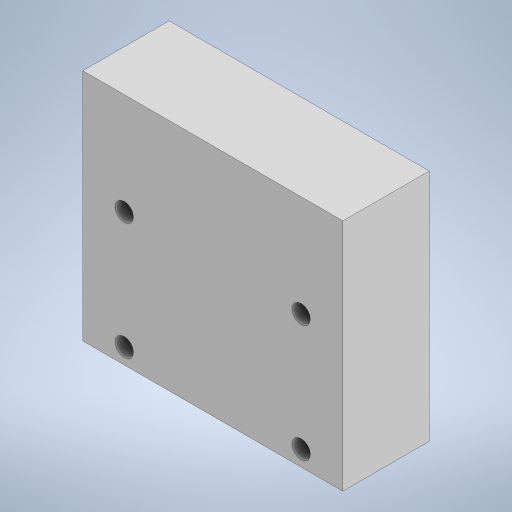
# Autodesk Inventor part: SUSTAINA-AUDIO-BOARD
Saved by Autodesk Inventor 2024.2 (Build 282272000, 272)
## iProperties
Created: 2024-06-01
Part Number: SUSTAINA-AUDIO-BOARD
Material: Generic
Document SubType Name: Modeling
Designer: Masato Kubotera
Density: 1 g/cm^3
Appearance: Default
Author: Masato Kubotera
Autodesk Inventor part; units mm, degrees
ref_plane "YZ Plane" through (0, 0, 0) normal (1, 0, 0) x (0, 1, 0)
ref_plane "XZ Plane" through (0, 0, 0) normal (0, 1, 0) x (-1, 0, 0)
ref_plane "XY Plane" through (0, 0, 0) normal (0, 0, 1) x (1, 0, 0)
sketch "Sketch1" plane through (0, 0, 0) normal (1, 0, 0) x (0, 1, 0)
  line L0 (-25, 22.5) -> (25, 22.5)
  line L1 (25, 22.5) -> (25, -22.5)
  line L2 (25, -22.5) -> (-25, -22.5)
  line L3 (-25, -22.5) -> (-25, 22.5)
  line L4 (-25, 22.5) -> (25, -22.5) construction
  line L5 (25, 22.5) -> (-25, -22.5) construction
  line L6 (-17, 3) -> (17, 3) construction
  line L7 (17, 3) -> (17, -19.5) construction
  line L8 (17, -19.5) -> (-17, -19.5) construction
  line L9 (-17, -19.5) -> (-17, 3) construction
  line L10 (-17, 3) -> (17, -19.5) construction
  line L11 (17, 3) -> (-17, -19.5) construction
  line L12 (0, 22.5) -> (0, -22.5) construction
  point P0 (0, 0)
  point P1 (0, -8.25)
  dimension "d0" = 50
  dimension "d1" = 45
  dimension "d2" = 34
  dimension "d3" = 22.5
  dimension "d4" = 3
  constraints: 26 end point, 6 midpoint, 4 coincident, 4 parallel, 2 horizontal, 2 perpendicular, 1 point on line
  measures "d0" distance of L1.end L2.end
  measures "d1" distance of L0.end L1.end
  measures "d2" distance of L7.end L8.end
  measures "d3" distance of L6.end L7.end
  measures "d4" distance between parallel lines of L2 L8
extrude "Extrusion1" add sketch "Sketch1" along normal blind 16.6
hole "Hole1" at (0, -17, 3) at (0, -17, -19.5) at (0, 17, -19.5) at (0, 17, 3) direction (1, 0, 0) diameter 3.5 end through all
body "Solid1"
